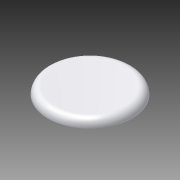
# Autodesk Inventor part: Frisbee
Saved by Autodesk Inventor 2013 (Build 170138000, 138)
## iProperties
Created: 2013-01-21
Part Number: Frisbee
Material: Glass
Document SubType Name: Modeling
Designer: Naphat
Density: 2.18 g/cm^3
Mass: 394.244 g
Surface Area: 1446.09 cm^2
Volume: 180.846 cm^3
Author: Naphat
Autodesk Inventor part; units mm, degrees
ref_plane "YZ Plane" through (0, 0, 0) normal (1, 0, 0) x (0, 1, 0)
ref_plane "XZ Plane" through (0, 0, 0) normal (0, 1, 0) x (-1, 0, 0)
ref_plane "XY Plane" through (0, 0, 0) normal (0, 0, 1) x (1, 0, 0)
sketch "Sketch1" plane through (0, 0, 0) normal (0, 1, 0) x (-1, 0, 0)
  circle A0 centre (0, 0) radius 138.938
  dimension "d0" = 277.876
  constraints: 1 centre point, 1 coincident
  measures "d0" diameter of A0
extrude "Extrusion1" add sketch "Sketch1" along normal blind 25.4
fillet "Fillet1" radius 25.4 1 edges at (138.938, 25.4, 0)
shell "Shell1" thickness 2.54 removed faces 2 at (78.7519, 0.0001, -114.4636) at (28.4576, 0, -60.367)
body "Solid1"
